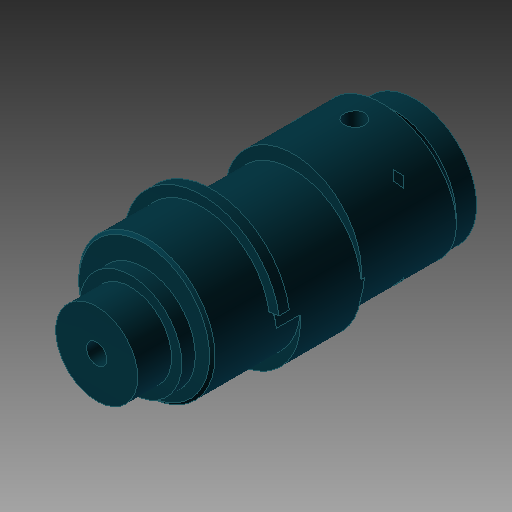
# Autodesk Inventor part: tri_ecc_cam
Saved by Autodesk Inventor 2017 (Build 210142000, 142)
## iProperties
Created: 2019-06-03
Part Number: tri_ecc_cam
Material: Generic
Document SubType Name: Modeling
Designer: paulg
Density: 1 g/cm^3
Appearance: Cadet Blue
Author: paulg
Autodesk Inventor part; units mm, degrees
ref_plane "YZ Plane" through (0, 0, 0) normal (1, 0, 0) x (0, 1, 0)
ref_plane "XY Plane" through (0, 0, 0) normal (0, 0, 1) x (1, 0, 0)
sketch "Sketch1" plane through (0, 0, 0) normal (0, 0, 1) x (1, 0, 0)
  line L0 (0, 0) -> (0, 1)
  circle A0 centre (0, 1) radius 10.05
  circle A1 centre (0, 0) radius 1.5
  dimension "d0" = 3
  dimension "d1" = 1
  dimension "d2" = 20.1
  constraints: 2 centre point, 2 coincident, 2 end point, 1 vertical
  measures "d0" diameter of A1
  measures "d1" distance of L0.start L0.end
  measures "d2" diameter of A0
extrude "Extrusion1" add sketch "Sketch1" along normal blind 18
sketch "Sketch2" plane through (0, 1, 18) normal (0, 0, 1) x (1, 0, 0)
  circle A0 centre (0, -1) radius 1.5 projected
  circle A1 centre (0, 0) radius 10.05 projected
  line L0 (0, -1) -> (0, -2)
  circle A2 centre (0, -2) radius 10.05
  dimension "d5" = 1
  constraints: 2 end point, 1 centre point, 1 coincident, 1 equal radius, 1 vertical
  measures "d5" distance of L0.start L0.end
extrude "Extrusion2" add sketch "Sketch2" along normal blind 13 contours A2 A1 | A1 A2 picked at (6.9861, -0.2008) picked at (1.0636, -10.6071)
sketch "Sketch3" plane through (0, -1, 31) normal (0, 0, 1) x (1, 0, 0)
  circle A0 centre (0, 1) radius 1.5 projected
  circle A1 centre (0, 0) radius 10.05 projected
  line L0 (0, 1) -> (0, 2)
  circle A2 centre (0, 2) radius 10.05
  dimension "d8" = 1
  constraints: 2 end point, 1 centre point, 1 coincident, 1 equal radius, 1 vertical
  measures "d8" distance of L0.start L0.end
extrude "Extrusion3" add sketch "Sketch3" along normal blind 9 contours A2 A1 | A1 A2 picked at (-6.9861, 0.2008) picked at (1.0636, 10.6071)
sketch "Sketch5" plane through (0, 1, 31) normal (0, 0, 1) x (1, 0, 0)
  arc A0 (-10.0001, -1) -> (10.0001, -1) centre (0, 0) ccw projected
  arc A1 (-10.0001, -1) -> (10.0001, -1) centre (0, -2) ccw projected
  point P0 (0, -1)
extrude "Extrusion4" cut sketch "Sketch5" against normal blind 4
sketch "Sketch6" plane through (0, 1, 40) normal (0, 0, 1) x (1, 0, 0)
  circle A0 centre (0, -1) radius 1.5 projected
  circle A1 centre (0, 0) radius 10.05 projected
  circle A2 centre (0, -1) radius 6.05
  dimension "d23" = 12.1
  constraints: 1 centre point, 1 coincident
  measures "d23" diameter of A2
extrude "Extrusion5" add sketch "Sketch6" along normal blind 7 contours A2
sketch "Sketch7" plane through (0, 1, 0) normal (0, 0, -1) x (-1, 0, 0)
  circle A0 centre (0, -1) radius 1.5 projected
  circle A1 centre (0, 0) radius 10.05 projected
  circle A2 centre (0, -1) radius 3.175
  dimension "d26" = 6.35
  constraints: 1 centre point, 1 coincident
  measures "d26" diameter of A2
extrude "Extrusion6" cut sketch "Sketch7" against normal blind 22 contours A2
ref_plane "Work Plane2" through (0, 0, 0) normal (0, 1, 0) x (-1, 0, 0)
sketch "Sketch9" plane through (0, 0, 0) normal (0, 1, 0) x (-1, 0, 0)
  line L0 (3.175, 22) -> (-3.175, 22) projected
  line L1 (3.175, 0) -> (-3.175, 0) projected
  line L2 (0, 0) -> (0, 22) construction
  line L3 (-2.75, 7.4123) -> (-2.75, 10.5877)
  line L4 (-2.75, 10.5877) -> (0, 12.1754)
  line L5 (0, 12.1754) -> (2.75, 10.5877)
  line L6 (2.75, 10.5877) -> (2.75, 7.4123)
  line L7 (2.75, 7.4123) -> (0, 5.8246)
  line L8 (0, 5.8246) -> (-2.75, 7.4123)
  line L9 (10.05, 18) -> (-10.05, 18) projected
  point P0 (0, 9)
  point P1 (-10.0001, 18)
  point P2 (10.0001, 18)
  dimension "d30" = 5.5
  dimension "d48" = 9
  constraints: 14 end point, 1 midpoint, 1 point on line, 1 vertical, 13 other
  measures "d30" distance between parallel lines of L6 L3
  measures "d48" distance from line of point (0, 9) L9
extrude "Extrusion7" cut sketch "Sketch9" along normal blind 4.5
sketch "Sketch10" plane through (0, 0, 0) normal (0, 1, 0) x (-1, 0, 0)
  line L0 (-2.75, 10.5877) -> (-2.75, 7.4123) projected
  line L1 (0, 12.1754) -> (-2.75, 10.5877) projected
  line L2 (2.75, 10.5877) -> (0, 12.1754) projected
  line L3 (2.75, 7.4123) -> (2.75, 10.5877) projected
  line L4 (0, 5.8246) -> (2.75, 7.4123) projected
  line L5 (-2.75, 7.4123) -> (0, 5.8246) projected
  line L6 (-2.75, 11.4123) -> (0, 9.8246) projected
  line L7 (-2.75, 14.5877) -> (-2.75, 11.4123) projected
  line L8 (0, 16.1754) -> (-2.75, 14.5877) projected
  line L9 (2.75, 14.5877) -> (0, 16.1754) projected
  line L10 (2.75, 11.4123) -> (2.75, 14.5877) projected
  line L11 (0, 9.8246) -> (2.75, 11.4123) projected
  line L12 (0, 5.8246) -> (2.75, 7.4123) projected
  line L13 (0, 5.8246) -> (0, 12.1754) construction
  line L14 (0, 16.1754) -> (0, 9.8246) construction
  point P0 (0, 0)
  point P1 (0, 13)
  point P2 (0, 9)
  constraints: 4 end point, 2 midpoint, 2 vertical
hole "Hole2" at (0, 0, 9) direction (0, 1, 0) diameter 3 end through all
sketch "Sketch11" plane through (0, 0, 0) normal (0, 1, 0) x (-1, 0, 0)
  line L0 (-10.0001, 18) -> (10.0001, 18) projected
  line L1 (10.0001, 18) -> (-10.0001, 18) projected
  line L2 (-10.05, 0) -> (10.05, 0) projected
  line L3 (7.5, -10) -> (-7.5, -10)
  line L4 (-7.5, -10) -> (-7.5, 10)
  line L5 (-7.5, 10) -> (7.5, 10)
  line L6 (7.5, 10) -> (7.5, -10)
  line L7 (7.5, -10) -> (-7.5, 10) construction
  line L8 (-7.5, -10) -> (7.5, 10) construction
  line L9 (-7.5, 9.2929) -> (-6.7929, 10)
  line L10 (-6.7929, 10) -> (-7.5, 10.7071)
  line L11 (-7.5, 10.7071) -> (-8.2071, 10)
  line L12 (-8.2071, 10) -> (-7.5, 9.2929)
  line L13 (-7.5, 9.2929) -> (-7.5, 10.7071) construction
  line L14 (-6.7929, 10) -> (-8.2071, 10) construction
  line L15 (7.5, 9.2929) -> (8.2071, 10)
  line L16 (8.2071, 10) -> (7.5, 10.7071)
  line L17 (7.5, 10.7071) -> (6.7929, 10)
  line L18 (6.7929, 10) -> (7.5, 9.2929)
  line L19 (7.5, 9.2929) -> (7.5, 10.7071) construction
  line L20 (8.2071, 10) -> (6.7929, 10) construction
  point P0 (0, 0)
  dimension "d42" = 8
  dimension "d43" = 1
  dimension "d44" = 1
  dimension "d45" = 15
  constraints: 36 end point, 6 midpoint, 6 parallel, 5 perpendicular, 3 horizontal, 1 other
  measures "d42" distance between parallel lines of L5 L0
  measures "d43" distance of L9.end L10.end
  measures "d44" distance of L10.end L11.end
  measures "d45" distance of L4.end L5.end
extrude "Extrusion8" cut sketch "Sketch11" along normal through all both and the other way through all contours L12 L11 L10 L5 L4 | L4 L5 L9 | L18 L5 L6 | L6 L5 L17 L16 L15
chamfer "Chamfer1" distance 0.4 angle 45 1 edges at (-10.05, 1, 40)
sketch "Sketch12" plane through (0, 1, 40) normal (0, 0, 1) x (1, 0, 0)
  circle A0 centre (0, -1) radius 6.05 projected
  circle A1 centre (0, 0) radius 9.65 projected
  circle A2 centre (0, -1) radius 1.5 projected
  circle A3 centre (0, -1) radius 7.55
  dimension "d52" = 1.5
  constraints: 1 centre point, 1 coincident
  measures "d52" radial gap between concentric circles of A0 A3
extrude "Extrusion9" add sketch "Sketch12" along normal blind 2 contours A3
sketch "Sketch14" plane through (0, 0, 0) normal (1, 0, 0) x (0, 1, 0)
  ellipse E0 centre (0, 12.1754) end of major axis (-3.175, 12.1754) minor radius 1.8331 (1.5869, 10.5877) -> (3.175, 12.1754) ccw projected
  line L0 (1.5869, 10.5877) -> (1.5869, 7.4123) projected
  ellipse E1 centre (0, 5.8246) end of major axis (3.175, 5.8246) minor radius 1.8331 (3.175, 5.8246) -> (1.5869, 7.4123) ccw projected
  ellipse E2 centre (0, 5.8246) end of major axis (3.175, 5.8246) minor radius 1.8331 (3.175, 5.8246) -> (1.5869, 7.4123) ccw projected
  line L1 (1.5869, 7.4123) -> (1.5869, 10.5877) projected
  ellipse E3 centre (0, 12.1754) end of major axis (-3.175, 12.1754) minor radius 1.8331 (1.5869, 10.5877) -> (3.175, 12.1754) ccw projected
  line L2 (3.175, 22) -> (-3.175, 22) projected
  line L3 (3.175, 0) -> (-3.175, 0) projected
  line L4 (3.175, 0) -> (-3.175, 0) projected
  line L5 (-9.05, 0) -> (11.05, 0) projected
  line L6 (-9.05, 3) -> (-13.05, 3)
  line L7 (-13.05, 3) -> (-13.05, 7)
  line L8 (-13.05, 7) -> (-9.05, 3)
  line L9 (-9.05, 0) -> (-13.05, 0)
  line L10 (-13.05, 0) -> (-13.05, 3)
  line L11 (-13.05, 3) -> (-9.05, 3)
  line L12 (-9.05, 3) -> (-9.05, 0)
  line L13 (0, -4.4) -> (0, 26.4) projected
  point P0 (0, 0)
  dimension "d55" = 4
  dimension "d56" = 4
  dimension "d57" = 3
  constraints: 14 end point, 2 horizontal, 2 parallel, 2 perpendicular, 1 collinear, 4 other
  measures "d55" distance of L6.start L6.end
  measures "d56" distance of L6.end L7.end
  measures "d57" distance of L9.end L10.end
revolve "Revolution1" cut sketch "Sketch14" angle 360 about axis through (0, 0, -10) along (0, 0, 1)
chamfer "Chamfer2" distance 1.6 angle 45 1 edges at (-1.5, 0, 22)
chamfer "Chamfer3" distance 0.5 angle 45 1 edges at (0, 9.05, 31)
chamfer "Chamfer4" distance 0.5 angle 45 1 edges at (0, -9.05, 18)
sketch "Sketch15" plane through (0, -1, 31) normal (0, 0, -1) x (-1, 0, 0)
  arc A0 (9.9258, 3.575) -> (-9.9258, 3.575) centre (0, 0) ccw projected
  arc A1 (9.9258, 3.575) -> (-9.9258, 3.575) centre (0, 2) ccw projected
  arc A2 (11.4073, 3.8101) -> (-11.4073, 3.8101) centre (0, 2) ccw
  line L0 (-9.9258, 3.575) -> (-11.4073, 3.8101)
  line L1 (9.9258, 3.575) -> (11.4073, 3.8101)
  point P0 (0, 1)
  dimension "d68" = 1.5
  constraints: 4 end point, 2 line through centre, 2 point on circle, 1 centre point
  measures "d68" radial gap between concentric circles of A1 A2
extrude "Extrusion10" add sketch "Sketch15" along normal blind 1 and the other way blind 0.5 contours A1 L0 A2 L1
equation "\"d44\" = d43"
body "Solid1"
